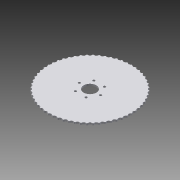
# Autodesk Inventor part: Big Sprocket
Saved by Autodesk Inventor 2015 (Build 190159000, 159)
## iProperties
Created: 2015-02-07
Part Number: Big Sprocket
Material: Aluminum 6061
Document SubType Name: Modeling
Designer: pltwe4
Density: 2.7 g/cm^3
Appearance: Aluminum - Flat
Author: pltwe4
Autodesk Inventor part; units mm, degrees
ref_plane "YZ Plane" through (0, 0, 0) normal (1, 0, 0) x (0, 1, 0)
ref_plane "XZ Plane" through (0, 0, 0) normal (0, 1, 0) x (-1, 0, 0)
ref_plane "XY Plane" through (0, 0, 0) normal (0, 0, 1) x (1, 0, 0)
sketch "Sketch1" plane through (0, 0, 0) normal (0, 1, 0) x (-1, 0, 0)
  circle A0 centre (0, 0) radius 93.98
  circle A1 centre (0, 0) radius 91.44 construction
  circle A2 centre (0, 0) radius 14.2812
  circle A3 centre (0, 0) radius 23.8125 construction
  circle A4 centre (23.8125, 0) radius 2.6162
  line L0 (0, -131.572) -> (0, 131.572) construction
  line L1 (-131.572, 0) -> (131.572, 0) construction
  circle A5 centre (11.9063, 20.6222) radius 2.6162
  circle A6 centre (-11.9062, 20.6222) radius 2.6162
  circle A7 centre (-23.8125, 0) radius 2.6162
  circle A8 centre (-11.9063, -20.6222) radius 2.6162
  circle A9 centre (11.9062, -20.6222) radius 2.6162
  line L2 (0, 0) -> (93.98, 0) construction
  line L3 (0, 0) -> (91.2491, 22.4909) construction
  line L4 (0, 0) -> (83.2152, 43.6747) construction
  line L5 (0, 0) -> (70.345, 62.3203) construction
  line L6 (0, 0) -> (53.3867, 77.344) construction
  line L7 (0, 0) -> (33.3258, 87.8728) construction
  line L8 (0, 0) -> (11.328, 93.2948) construction
  line L9 (0, 0) -> (-11.328, 93.2948) construction
  line L10 (0, 0) -> (-33.3258, 87.8728) construction
  line L11 (0, 0) -> (-53.3867, 77.344) construction
  line L12 (0, 0) -> (-70.345, 62.3203) construction
  line L13 (0, 0) -> (-83.2152, 43.6747) construction
  line L14 (0, 0) -> (-91.2491, 22.4909) construction
  line L15 (0, 0) -> (-93.98, 0) construction
  line L16 (0, 0) -> (-91.2491, -22.4909) construction
  line L17 (0, 0) -> (-83.2152, -43.6747) construction
  line L18 (0, 0) -> (-70.345, -62.3203) construction
  line L19 (0, 0) -> (-53.3867, -77.344) construction
  line L20 (0, 0) -> (-33.3258, -87.8728) construction
  line L21 (0, 0) -> (-11.328, -93.2948) construction
  line L22 (0, 0) -> (11.328, -93.2948) construction
  line L23 (0, 0) -> (33.3258, -87.8728) construction
  line L24 (0, 0) -> (53.3867, -77.344) construction
  line L25 (0, 0) -> (70.345, -62.3203) construction
  line L26 (0, 0) -> (83.2152, -43.6747) construction
  line L27 (0, 0) -> (91.2491, -22.4909) construction
  dimension "d0" = 187.96
  dimension "d3" = 47.625
  dimension "d1" = 182.88
  dimension "d2" = 28.5623
  dimension "d4" = 5.2324
  dimension "d7" = 360
  dimension "d11" = 360
  constraints: 52 end point, 8 centre point, 4 coincident, 2 horizontal alignment, 2 point on line, 96 other
  measures "d1" diameter of A1
  measures "d2" diameter of A2
  measures "d4" diameter of A4
extrude "Extrusion1" add sketch "Sketch1" along normal blind 3.9624 contours A0 | A4 | A5 | A6 | A7 | A8 | A9
sketch "Sketch2" plane through (0, 3.9624, 0) normal (0, 1, 0) x (1, 0, 0)
  circle A0 centre (0, 0) radius 14.2812 projected
  circle A1 centre (0, 0) radius 93.98 projected
  line L0 (0, 0) -> (0, 93.98) construction
  line L1 (0, 0) -> (-9.8236, 93.4652) construction
  line L2 (0, 0) -> (-19.5395, 91.9263) construction
  line L3 (0, 0) -> (-29.0414, 89.3803) construction
  line L4 (0, 0) -> (-38.2251, 85.855) construction
  line L5 (0, 0) -> (-46.99, 81.3891) construction
  line L6 (0, 0) -> (-55.2401, 76.0314) construction
  line L7 (0, 0) -> (-62.8849, 69.8408) construction
  line L8 (0, 0) -> (-69.8408, 62.8849) construction
  line L9 (0, 0) -> (-76.0314, 55.2401) construction
  line L10 (0, 0) -> (-81.3891, 46.99) construction
  line L11 (0, 0) -> (-85.855, 38.2251) construction
  line L12 (0, 0) -> (-89.3803, 29.0414) construction
  line L13 (0, 0) -> (-91.9263, 19.5395) construction
  line L14 (0, 0) -> (-93.4652, 9.8236) construction
  line L15 (0, 0) -> (-93.98, 0) construction
  line L16 (0, 0) -> (-93.4652, -9.8236) construction
  line L17 (0, 0) -> (-91.9263, -19.5395) construction
  line L18 (0, 0) -> (-89.3803, -29.0414) construction
  line L19 (0, 0) -> (-85.855, -38.2251) construction
  line L20 (0, 0) -> (-81.3891, -46.99) construction
  line L21 (0, 0) -> (-76.0314, -55.2401) construction
  line L22 (0, 0) -> (-69.8408, -62.8849) construction
  line L23 (0, 0) -> (-62.8849, -69.8408) construction
  line L24 (0, 0) -> (-55.2401, -76.0314) construction
  line L25 (0, 0) -> (-46.99, -81.3891) construction
  line L26 (0, 0) -> (-38.2251, -85.855) construction
  line L27 (0, 0) -> (-29.0414, -89.3803) construction
  line L28 (0, 0) -> (-19.5395, -91.9263) construction
  line L29 (0, 0) -> (-9.8236, -93.4652) construction
  line L30 (0, 0) -> (0, -93.98) construction
  line L31 (0, 0) -> (9.8236, -93.4652) construction
  line L32 (0, 0) -> (19.5395, -91.9263) construction
  line L33 (0, 0) -> (29.0414, -89.3803) construction
  line L34 (0, 0) -> (38.2251, -85.855) construction
  line L35 (0, 0) -> (46.99, -81.3891) construction
  line L36 (0, 0) -> (55.2401, -76.0314) construction
  line L37 (0, 0) -> (62.8849, -69.8408) construction
  line L38 (0, 0) -> (69.8408, -62.8849) construction
  line L39 (0, 0) -> (76.0314, -55.2401) construction
  line L40 (0, 0) -> (81.3891, -46.99) construction
  line L41 (0, 0) -> (85.855, -38.2251) construction
  line L42 (0, 0) -> (89.3803, -29.0414) construction
  line L43 (0, 0) -> (91.9263, -19.5395) construction
  line L44 (0, 0) -> (93.4652, -9.8236) construction
  line L45 (0, 0) -> (93.98, 0) construction
  line L46 (0, 0) -> (93.4652, 9.8236) construction
  line L47 (0, 0) -> (91.9263, 19.5395) construction
  line L48 (0, 0) -> (89.3803, 29.0414) construction
  line L49 (0, 0) -> (85.855, 38.2251) construction
  line L50 (0, 0) -> (81.3891, 46.99) construction
  line L51 (0, 0) -> (76.0314, 55.2401) construction
  line L52 (0, 0) -> (69.8408, 62.8849) construction
  line L53 (0, 0) -> (62.8849, 69.8408) construction
  line L54 (0, 0) -> (55.2401, 76.0314) construction
  line L55 (0, 0) -> (46.99, 81.3891) construction
  line L56 (0, 0) -> (38.2251, 85.855) construction
  line L57 (0, 0) -> (29.0414, 89.3803) construction
  line L58 (0, 0) -> (19.5395, 91.9263) construction
  line L59 (0, 0) -> (9.8236, 93.4652) construction
  circle A2 centre (0, 0) radius 91.44 construction
  line L60 (0, 0) -> (4.9185, 93.8512) construction
  circle A3 centre (0, 0) radius 93.98 construction
  arc A4 (1.5833, 93.1344) -> (8.1606, 92.7897) centre (5.0008, 95.421) ccw
  circle A5 centre (0, 0) radius 93.98 construction
  line L61 (138.205, 0) -> (-138.2655, 0) construction
  arc A6 (9.8236, 93.4652) -> (8.1606, 92.7897) centre (9.6245, 91.5706) ccw
  arc A7 (1.5833, 93.1344) -> (0, 93.98) centre (0, 92.075) ccw
  arc A8 (9.8236, 93.4652) -> (0, 93.98) centre (0, 0) ccw
  arc A9 (-9.8236, 93.4652) -> (19.5395, 91.9263) centre (0, 0) ccw
  dimension "d32" = 182.88
  dimension "d35" = 1.905
  dimension "d36" = 1.905
  dimension "d37" = 4.112
  constraints: 122 end point, 14 point on circle, 6 centre point, 3 point on line, 2 coincident, 1 perpendicular, 1 tangent, 184 other
  measures "d32" diameter of A2
  measures "d35" radius of A7
  measures "d36" radius of A6
  measures "d37" radius of A4
extrude "Extrusion3" cut sketch "Sketch2" against normal up to next contours A6 A4 A7 A1 picked at (4.8737, 92.9962)
pattern_circular "Circular Pattern4" count 60 over 360 about axis through (0, 0, 0) along (0, 1, 0) of "Extrusion3"
extrude "Extrusion4" cut sketch "Sketch1" along normal up to next contours A4 | A5 | A6 | A7 | A8 | A9
body "Solid1"
